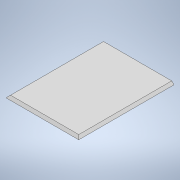
# Autodesk Inventor part: predni blatnik
Saved by Autodesk Inventor 2022 (Build 260153000, 153)
## iProperties
Created: 2022-12-25
Part Number: predni blatnik
Material: Všeobecné
Document SubType Name: Modeling
Designer: matys
Density: 1 g/cm^3
Appearance: Výchozí
Author: matys
Autodesk Inventor part; units mm, degrees
ref_plane "YZ Plane" through (0, 0, 0) normal (1, 0, 0) x (0, 1, 0)
ref_plane "XZ Plane" through (0, 0, 0) normal (0, 1, 0) x (-1, 0, 0)
ref_plane "XY Plane" through (0, 0, 0) normal (0, 0, 1) x (1, 0, 0)
sketch "Sketch1" plane through (0, 0, 0) normal (0, 1, 0) x (-1, 0, 0)
  line L0 (0, 0) -> (0, -41.9)
  line L1 (0, -41.9) -> (32, -41.9)
  line L2 (32, -41.9) -> (32, 0)
  line L3 (32, 0) -> (0, 0)
  dimension "d0" = 41.9
  dimension "d1" = 32
  constraints: 8 end point, 3 perpendicular, 1 vertical
  measures "d0" distance of L0.start L0.end
  measures "d1" distance of L0.end L1.end
extrude "Extrusion1" add sketch "Sketch1" along normal blind 1
chamfer "Chamfer1" distance 1 angle 45 3 edges at (-16, 1, 0) (0, 1, -20.95) (-32, 1, -20.95)
body "Solid1"
